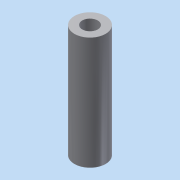
# Autodesk Inventor part: magnet_spacer
Saved by Autodesk Inventor 2014 (Build 180170000, 170)
## iProperties
Created: 2014-04-24
Part Number: magnet_spacer
Material: Aluminum 6061
Document SubType Name: Modeling
Designer: RDavis
Density: 2.71 g/cm^3
Appearance: Aluminum - Flat
Author: RDavis
Autodesk Inventor part; units mm, degrees
ref_plane "YZ Plane" through (0, 0, 0) normal (1, 0, 0) x (0, 1, 0)
ref_plane "XZ Plane" through (0, 0, 0) normal (0, 1, 0) x (-1, 0, 0)
ref_plane "XY Plane" through (0, 0, 0) normal (0, 0, 1) x (1, 0, 0)
sketch "Sketch1" plane through (0, 0, 0) normal (0, 0, 1) x (1, 0, 0)
  circle A0 centre (0, 0) radius 1.5875
  circle A1 centre (0, 0) radius 3.175
  dimension "d0" = 3.175
  dimension "d1" = 6.35
  constraints: 2 centre point, 2 coincident
  measures "d0" diameter of A0
  measures "d1" diameter of A1
extrude "Extrusion1" add sketch "Sketch1" along normal mid plane 23
body "Solid1"
